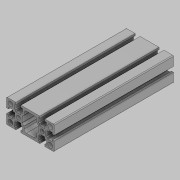
# Autodesk Inventor part: AFS-3060-200
Saved by Autodesk Inventor 2021.2 (Build 252289000, 289)
## iProperties
Created: 2016-10-06
Part Number: AFS-3060-200
Material: Generic
Document SubType Name: Modeling
Designer: gisen
Density: 1 g/cm^3
Appearance: Default
Sending System: Autodesk Inventor 2014
Preprocessor: ST-DEVELOPER v15.2
Title: C:\Users\AMS43\Documents\Inventor\AMS\misumi\フレーム_ipt\フレーム_stp\AFS-3060-6.ipt.stp
Author: AMS43
Autodesk Inventor part; units mm, degrees
ref_plane "YZ Plane" through (0, 0, 0) normal (1, 0, 0) x (0, 1, 0)
ref_plane "XZ Plane" through (0, 0, 0) normal (0, 1, 0) x (-1, 0, 0)
ref_plane "XY Plane" through (0, 0, 0) normal (0, 0, 1) x (1, 0, 0)
feature "ソリッド1" [suppressed]
sketch "スケッチ2" plane through (0, 0, 0) normal (0, 0, 1) x (1, 0, 0)
  line L0 (9.85, -12.5) -> (9.85, -7) projected
  line L1 (9.85, -7) -> (11.85, -7) projected
  line L2 (11.85, -7) -> (11.85, -4.5) projected
  line L3 (11.85, -4.5) -> (18.15, -4.5) projected
  line L4 (18.15, -4.5) -> (18.15, -7) projected
  line L5 (18.15, -7) -> (20.15, -7) projected
  line L6 (20.15, -7) -> (20.15, -12.5) projected
  line L7 (20.15, -12.5) -> (18.15, -12.5) projected
  line L8 (18.15, -12.5) -> (18.15, -15) projected
  line L9 (18.15, -15) -> (29, -15) projected
  arc A0 (29, -15) -> (30, -14) centre (29, -14) ccw projected
  line L10 (30, -14) -> (30, -3.15) projected
  line L11 (30, -3.15) -> (27.5, -3.15) projected
  line L12 (27.5, -3.15) -> (27.5, -5.15) projected
  line L13 (27.5, -5.15) -> (22, -5.15) projected
  line L14 (22, -5.15) -> (22, -3.15) projected
  line L15 (22, -3.15) -> (19.5, -3.15) projected
  line L16 (19.5, -3.15) -> (19.5, 3.15) projected
  line L17 (19.5, 3.15) -> (22, 3.15) projected
  line L18 (22, 3.15) -> (22, 5.15) projected
  line L19 (22, 5.15) -> (27.5, 5.15) projected
  line L20 (27.5, 5.15) -> (27.5, 3.15) projected
  line L21 (27.5, 3.15) -> (30, 3.15) projected
  line L22 (30, 3.15) -> (30, 14) projected
  arc A1 (30, 14) -> (29, 15) centre (29, 14) ccw projected
  line L23 (29, 15) -> (18.15, 15) projected
  line L24 (18.15, 15) -> (18.15, 12.5) projected
  line L25 (18.15, 12.5) -> (20.15, 12.5) projected
  line L26 (20.15, 12.5) -> (20.15, 7) projected
  line L27 (20.15, 7) -> (18.15, 7) projected
  line L28 (18.15, 7) -> (18.15, 4.5) projected
  line L29 (18.15, 4.5) -> (11.85, 4.5) projected
  line L30 (11.85, 4.5) -> (11.85, 7) projected
  line L31 (11.85, 7) -> (9.85, 7) projected
  line L32 (9.85, 7) -> (9.85, 12.5) projected
  line L33 (9.85, 12.5) -> (11.85, 12.5) projected
  line L34 (11.85, 12.5) -> (11.85, 15) projected
  line L35 (11.85, 15) -> (-11.85, 15) projected
  line L36 (-11.85, 15) -> (-11.85, 12.5) projected
  line L37 (-11.85, 12.5) -> (-9.85, 12.5) projected
  line L38 (-9.85, 12.5) -> (-9.85, 7) projected
  line L39 (-9.85, 7) -> (-11.85, 7) projected
  line L40 (-11.85, 7) -> (-11.85, 4.5) projected
  line L41 (-11.85, 4.5) -> (-18.15, 4.5) projected
  line L42 (-18.15, 4.5) -> (-18.15, 7) projected
  line L43 (-18.15, 7) -> (-20.15, 7) projected
  line L44 (-20.15, 7) -> (-20.15, 12.5) projected
  line L45 (-20.15, 12.5) -> (-18.15, 12.5) projected
  line L46 (-18.15, 12.5) -> (-18.15, 15) projected
  line L47 (-18.15, 15) -> (-29, 15) projected
  arc A2 (-29, 15) -> (-30, 14) centre (-29, 14) ccw projected
  line L48 (-30, 14) -> (-30, 3.15) projected
  line L49 (-30, 3.15) -> (-27.5, 3.15) projected
  line L50 (-27.5, 3.15) -> (-27.5, 5.15) projected
  line L51 (-27.5, 5.15) -> (-22, 5.15) projected
  line L52 (-22, 5.15) -> (-22, 3.15) projected
  line L53 (-22, 3.15) -> (-19.5, 3.15) projected
  line L54 (-19.5, 3.15) -> (-19.5, -3.15) projected
  line L55 (-19.5, -3.15) -> (-22, -3.15) projected
  line L56 (-22, -3.15) -> (-22, -5.15) projected
  line L57 (-22, -5.15) -> (-27.5, -5.15) projected
  line L58 (-27.5, -5.15) -> (-27.5, -3.15) projected
  line L59 (-27.5, -3.15) -> (-30, -3.15) projected
  line L60 (-30, -3.15) -> (-30, -14) projected
  arc A3 (-30, -14) -> (-29, -15) centre (-29, -14) ccw projected
  line L61 (-29, -15) -> (-18.15, -15) projected
  line L62 (-18.15, -15) -> (-18.15, -12.5) projected
  line L63 (-18.15, -12.5) -> (-20.15, -12.5) projected
  line L64 (-20.15, -12.5) -> (-20.15, -7) projected
  line L65 (-20.15, -7) -> (-18.15, -7) projected
  line L66 (-18.15, -7) -> (-18.15, -4.5) projected
  line L67 (-18.15, -4.5) -> (-11.85, -4.5) projected
  line L68 (-11.85, -4.5) -> (-11.85, -7) projected
  line L69 (-11.85, -7) -> (-9.85, -7) projected
  line L70 (-9.85, -7) -> (-9.85, -12.5) projected
  line L71 (-9.85, -12.5) -> (-11.85, -12.5) projected
  line L72 (-11.85, -12.5) -> (-11.85, -15) projected
  line L73 (-11.85, -15) -> (11.85, -15) projected
  line L74 (11.85, -15) -> (11.85, -12.5) projected
  line L75 (11.85, -12.5) -> (9.85, -12.5) projected
  arc A4 (-8, -9) -> (-5, -12) centre (-5, -9) ccw projected
  line L76 (-8, -9) -> (-8, -6.2071) projected
  arc A5 (-8, -6.2071) -> (-8.1464, -5.8536) centre (-8.5, -6.2071) ccw projected
  line L77 (-8.1464, -5.8536) -> (-10.3536, -3.6464) projected
  arc A6 (-10.5, -3.2929) -> (-10.3536, -3.6464) centre (-10, -3.2929) ccw projected
  line L78 (-10.5, -3.2929) -> (-10.5, 3.2929) projected
  arc A7 (-10.3536, 3.6464) -> (-10.5, 3.2929) centre (-10, 3.2929) ccw projected
  line L79 (-10.3536, 3.6464) -> (-8.1464, 5.8536) projected
  arc A8 (-8.1464, 5.8536) -> (-8, 6.2071) centre (-8.5, 6.2071) ccw projected
  line L80 (-8, 6.2071) -> (-8, 9) projected
  arc A9 (-5, 12) -> (-8, 9) centre (-5, 9) ccw projected
  line L81 (-5, 12) -> (5, 12) projected
  arc A10 (8, 9) -> (5, 12) centre (5, 9) ccw projected
  line L82 (8, 9) -> (8, 6.2071) projected
  arc A11 (8, 6.2071) -> (8.1464, 5.8536) centre (8.5, 6.2071) ccw projected
  line L83 (8.1464, 5.8536) -> (10.3536, 3.6464) projected
  arc A12 (10.5, 3.2929) -> (10.3536, 3.6464) centre (10, 3.2929) ccw projected
  line L84 (10.5, 3.2929) -> (10.5, -3.2929) projected
  arc A13 (10.3536, -3.6464) -> (10.5, -3.2929) centre (10, -3.2929) ccw projected
  line L85 (10.3536, -3.6464) -> (8.1464, -5.8536) projected
  arc A14 (8.1464, -5.8536) -> (8, -6.2071) centre (8.5, -6.2071) ccw projected
  line L86 (8, -6.2071) -> (8, -9) projected
  arc A15 (5, -12) -> (8, -9) centre (5, -9) ccw projected
  line L87 (5, -12) -> (-5, -12) projected
  circle A16 centre (25, 10) radius 3 projected
  circle A17 centre (-25, -10) radius 3 projected
  circle A18 centre (-25, 10) radius 3 projected
  circle A19 centre (25, -10) radius 3 projected
  circle A20 centre (15, 0) radius 2.5 projected
  circle A21 centre (-15, 0) radius 2.5 projected
  point P0 (0, 0)
extrude "押し出し1" add sketch "スケッチ2" along normal blind 150
equation "\"d1\" = L"
equation "\"L\" = 150"
